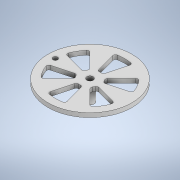
# Autodesk Inventor part: trục quay
Saved by Autodesk Inventor 2020 (Build 240168000, 168)
## iProperties
Created: 2022-11-23
Part Number: trục quay
Material: Generic
Document SubType Name: Modeling
Designer: ADMIN
Density: 1 g/cm^3
Appearance: Default
Author: ADMIN
Autodesk Inventor part; units mm, degrees
ref_plane "YZ Plane" through (0, 0, 0) normal (1, 0, 0) x (0, 1, 0)
ref_plane "XZ Plane" through (0, 0, 0) normal (0, 1, 0) x (-1, 0, 0)
ref_plane "XY Plane" through (0, 0, 0) normal (0, 0, 1) x (1, 0, 0)
sketch "Sketch1" plane through (0, 0, 0) normal (0, 1, 0) x (-1, 0, 0)
  circle A0 centre (0, 0) radius 4
  dimension "d0" = 8
  constraints: 1 centre point, 1 coincident
  measures "d0" diameter of A0
extrude "Extrusion1" add sketch "Sketch1" along normal blind 15
sketch "Sketch2" plane through (0, 15, 0) normal (0, 1, 0) x (1, 0, 0)
  circle A0 centre (0, 0) radius 3
  dimension "d3" = 6
  constraints: 1 centre point, 1 coincident
  measures "d3" diameter of A0
extrude "Extrusion2" cut sketch "Sketch2" against normal blind 13
sketch "Sketch3" plane through (0, 0, 0) normal (1, 0, 0) x (0, 1, 0)
  line L0 (15, -4) -> (15, 4) projected
  circle A0 centre (4, 0) radius 2
  line L1 (0, -4) -> (0, 4) projected
  point P0 (0, 0)
  dimension "d8" = 4
  dimension "d9" = 4
  constraints: 1 centre point
  measures "d8" diameter of A0
  measures "d9" distance from line of L1 A0.centre
extrude "Extrusion3" cut sketch "Sketch3" against normal blind 25
sketch "Sketch9" plane through (0, 15, 0) normal (0, 1, 0) x (1, 0, 0)
  circle A0 centre (0, 0) radius 40
  dimension "d47" = 80
  constraints: 1 centre point, 1 coincident
  measures "d47" diameter of A0
extrude "Extrusion8" add sketch "Sketch9" along normal blind 4
sketch "Sketch10" plane through (0, 19, 0) normal (0, 1, 0) x (1, 0, 0)
  circle A0 centre (0, 0) radius 3
  circle A1 centre (-33, 0) radius 2.25
  circle A2 centre (0, 0) radius 3 projected
  line L0 (0, 0) -> (-40, 0)
  circle A3 centre (0, 0) radius 4 projected
  arc A4 (-31.2581, -10.5797) -> (-24.7914, -21.7805) centre (0, 0) ccw
  arc A5 (-29.8813, -8.0067) -> (-31.2581, -10.5797) centre (-29.3637, -9.9385) ccw
  arc A6 (-24.7914, -21.7805) -> (-21.8746, -21.8746) centre (-23.2889, -20.4604) ccw
  arc A7 (-9.0928, -4.1619) -> (-8.1507, -5.7937) centre (0, 0) ccw
  line L1 (-8.3666, -8.3666) -> (-21.8746, -21.8746)
  line L2 (-11.429, -3.0624) -> (-29.8813, -8.0067)
  arc A8 (-8.3666, -8.3666) -> (-8.1507, -5.7937) centre (-9.7808, -6.9524) ccw
  arc A9 (-9.0928, -4.1619) -> (-11.429, -3.0624) centre (-10.9114, -4.9942) ccw
  arc A10 (-6.4667, -32.3602) -> (6.4667, -32.3602) centre (0, 0) ccw
  line L3 (-3.0624, -11.429) -> (-8.0067, -29.8813)
  arc A11 (-0.9421, -9.9555) -> (-3.0624, -11.429) centre (-1.1305, -11.9466) ccw
  line L4 (3.0624, -11.429) -> (8.0067, -29.8813)
  arc A12 (-0.9421, -9.9555) -> (0.9421, -9.9555) centre (0, 0) ccw
  arc A13 (3.0624, -11.429) -> (0.9421, -9.9555) centre (1.1305, -11.9466) ccw
  arc A14 (6.4667, -32.3602) -> (8.0067, -29.8813) centre (6.0748, -30.399) ccw
  arc A15 (-8.0067, -29.8813) -> (-6.4667, -32.3602) centre (-6.0748, -30.399) ccw
  arc A16 (24.7914, -21.7805) -> (31.2581, -10.5797) centre (0, 0) ccw
  line L5 (8.3666, -8.3666) -> (21.8746, -21.8746)
  arc A17 (8.1507, -5.7937) -> (8.3666, -8.3666) centre (9.7808, -6.9524) ccw
  line L6 (11.429, -3.0624) -> (29.8813, -8.0067)
  arc A18 (8.1507, -5.7937) -> (9.0928, -4.1619) centre (0, 0) ccw
  arc A19 (11.429, -3.0624) -> (9.0928, -4.1619) centre (10.9114, -4.9942) ccw
  arc A20 (31.2581, -10.5797) -> (29.8813, -8.0067) centre (29.3637, -9.9385) ccw
  arc A21 (21.8746, -21.8746) -> (24.7914, -21.7805) centre (23.2889, -20.4604) ccw
  arc A22 (31.2581, 10.5797) -> (24.7914, 21.7805) centre (0, 0) ccw
  line L7 (11.429, 3.0624) -> (29.8813, 8.0067)
  arc A23 (9.0928, 4.1619) -> (11.429, 3.0624) centre (10.9114, 4.9942) ccw
  line L8 (8.3666, 8.3666) -> (21.8746, 21.8746)
  arc A24 (9.0928, 4.1619) -> (8.1507, 5.7937) centre (0, 0) ccw
  arc A25 (8.3666, 8.3666) -> (8.1507, 5.7937) centre (9.7808, 6.9524) ccw
  arc A26 (24.7914, 21.7805) -> (21.8746, 21.8746) centre (23.2889, 20.4604) ccw
  arc A27 (29.8813, 8.0067) -> (31.2581, 10.5797) centre (29.3637, 9.9385) ccw
  arc A28 (6.4667, 32.3602) -> (-6.4667, 32.3602) centre (0, 0) ccw
  line L9 (3.0624, 11.429) -> (8.0067, 29.8813)
  arc A29 (0.9421, 9.9555) -> (3.0624, 11.429) centre (1.1305, 11.9466) ccw
  line L10 (-3.0624, 11.429) -> (-8.0067, 29.8813)
  arc A30 (0.9421, 9.9555) -> (-0.9421, 9.9555) centre (0, 0) ccw
  arc A31 (-3.0624, 11.429) -> (-0.9421, 9.9555) centre (-1.1305, 11.9466) ccw
  arc A32 (-6.4667, 32.3602) -> (-8.0067, 29.8813) centre (-6.0748, 30.399) ccw
  arc A33 (8.0067, 29.8813) -> (6.4667, 32.3602) centre (6.0748, 30.399) ccw
  arc A34 (-24.7914, 21.7805) -> (-31.2581, 10.5797) centre (0, 0) ccw
  line L11 (-8.3666, 8.3666) -> (-21.8746, 21.8746)
  arc A35 (-8.1507, 5.7937) -> (-8.3666, 8.3666) centre (-9.7808, 6.9524) ccw
  line L12 (-11.429, 3.0624) -> (-29.8813, 8.0067)
  arc A36 (-8.1507, 5.7937) -> (-9.0928, 4.1619) centre (0, 0) ccw
  arc A37 (-11.429, 3.0624) -> (-9.0928, 4.1619) centre (-10.9114, 4.9942) ccw
  arc A38 (-31.2581, 10.5797) -> (-29.8813, 8.0067) centre (-29.3637, 9.9385) ccw
  arc A39 (-21.8746, 21.8746) -> (-24.7914, 21.7805) centre (-23.2889, 20.4604) ccw
  point P0 (-3, 0)
  point P1 (-31.8756, -8.541)
  point P2 (-23.3345, -23.3345)
  point P3 (-9.6593, -2.5882)
  point P4 (-7.0711, -7.0711)
  dimension "d54" = 4.5
  dimension "d62" = 2
  dimension "d63" = 2
  dimension "d66" = 360
  constraints: 76 point on circle, 37 centre point, 26 end point, 8 tangent, 3 coincident, 2 equal radius, 2 horizontal alignment, 2 point on line, 1 horizontal, 134 other
  measures "d54" diameter of A1
  measures "d62" radius of A5
  measures "d63" radius of A8
extrude "Extrusion9" cut sketch "Sketch10" against normal through all contours A0 | L0 A1 | A1 L0 | A5 L2 A9 A7 A8 L1 A6 A4 | A15 L3 A11 A12 A13 L4 A14 A10 | A21 L5 A17 A18 A19 L6 A20 A16 | A27 L7 A23 A24 A25 L8 A26 A22 | A33 L9 A29 A30 A31 L10 A32 A28 | A39 L11 A35 A36 A37 L12 A38 A34
body "Solid1"
